Autodesk Fusion 360 part; units mm, degrees
note: some values were not read from the file. Set by a fixed rule: which sketch regions a step uses.
(part 8 of 20)
  spline S42 degree 5 poles (20.11, 20.9575) (20.11, 20.9576) (20.1102, 20.9577) (20.1104, 20.958) (20.1107, 20.9583) (20.1112, 20.9589) (20.1118, 20.9595) (20.1125, 20.9602) (20.1132, 20.961) (20.114, 20.9619) (20.1149, 20.9629) (20.1159, 20.9639) (20.1169, 20.9651) (20.118, 20.9663) (20.1192, 20.9675) (20.1204, 20.9689) (20.1217, 20.9704) (20.123, 20.9719) (20.1245, 20.9735) (20.126, 20.9752) (20.1275, 20.9769) (20.1291, 20.9787) (20.1308, 20.9806) (20.1325, 20.9826) (20.1343, 20.9847) (20.1361, 20.9868) (20.138, 20.989) (20.1399, 20.9912) (20.1419, 20.9936) (20.144, 20.996) (20.1461, 20.9984) (20.1482, 21.001) (20.1504, 21.0036) (20.1527, 21.0063) (20.155, 21.009) (20.1573, 21.0119) (20.1597, 21.0148) (20.1622, 21.0177) (20.1647, 21.0207) (20.1672, 21.0238) (20.1698, 21.027) (20.1724, 21.0302) (20.1751, 21.0335) (20.1778, 21.0368) (20.1806, 21.0403) (20.1834, 21.0437) (20.1862, 21.0473) (20.1891, 21.0509) (20.192, 21.0546) (20.195, 21.0583) (20.198, 21.0621) (20.201, 21.066) (20.2041, 21.0699) (20.2072, 21.0739) (20.2103, 21.0779) (20.2135, 21.082) (20.2167, 21.0862) (20.22, 21.0904) (20.2233, 21.0947) (20.2266, 21.099) (20.23, 21.1034) (20.2333, 21.1079) (20.2368, 21.1124) (20.2402, 21.117) (20.2437, 21.1216) (20.2472, 21.1263) (20.2508, 21.1311) (20.2544, 21.1359) (20.258, 21.1408) (20.2616, 21.1457) (20.2653, 21.1507) (20.269, 21.1557) (20.2727, 21.1608) (20.2765, 21.166) (20.2802, 21.1712) (20.2841, 21.1764) (20.2879, 21.1818) (20.2918, 21.1871) (20.2956, 21.1926) (20.2996, 21.1981) (20.3035, 21.2036) (20.3075, 21.2092) (20.3115, 21.2148) (20.3155, 21.2205) (20.3195, 21.2263) (20.3236, 21.2321) (20.3277, 21.238) (20.3318, 21.2439) (20.3359, 21.2498) (20.3401, 21.2559) (20.3442, 21.2619) (20.3484, 21.2681) (20.3527, 21.2742) (20.3569, 21.2805) (20.3612, 21.2867) (20.3655, 21.2931) (20.3698, 21.2995) (20.3741, 21.3059) (20.3784, 21.3124) (20.3828, 21.3189) (20.3872, 21.3255) (20.3916, 21.3321) (20.396, 21.3388) (20.4004, 21.3455) (20.4049, 21.3523) (20.4094, 21.3592) (20.4139, 21.3661) (20.4184, 21.373) (20.4229, 21.38) (20.4274, 21.387) (20.432, 21.3941) (20.4366, 21.4012) (20.4412, 21.4084) (20.4458, 21.4156) (20.4504, 21.4229) (20.455, 21.4302) (20.4597, 21.4376) (20.4644, 21.445) (20.469, 21.4525) (20.4737, 21.46) (20.4784, 21.4676) (20.4832, 21.4752) (20.4879, 21.4828) (20.4927, 21.4905) (20.4974, 21.4983) (20.5022, 21.5061) (20.507, 21.5139) (20.5118, 21.5218) (20.5166, 21.5297) (20.5214, 21.5377) (20.5263, 21.5458) (20.5311, 21.5538) (20.536, 21.5619) (20.5409, 21.5701) (20.5457, 21.5783) (20.5506, 21.5866) (20.5555, 21.5949) (20.5605, 21.6032) (20.5654, 21.6116) (20.5703, 21.6201) (20.5753, 21.6285) (20.5802, 21.6371) (20.5852, 21.6456) (20.5902, 21.6542) (20.5951, 21.6629) (20.6001, 21.6716) (20.6051, 21.6803) (20.6101, 21.6891) (20.6152, 21.698) (20.6202, 21.7068) (20.6252, 21.7158) (20.6303, 21.7247) (20.6353, 21.7337) (20.6404, 21.7428) (20.6454, 21.7519) (20.6505, 21.761) (20.6556, 21.7702) (20.6607, 21.7794) (20.6658, 21.7887) (20.6709, 21.798) (20.676, 21.8073) (20.6811, 21.8167) (20.6862, 21.8261) (20.6913, 21.8356) (20.6965, 21.8451) (20.7016, 21.8547) (20.7067, 21.8643) (20.7119, 21.8739) (20.717, 21.8836) (20.7222, 21.8933) (20.7274, 21.9031) (20.7325, 21.9129) (20.7377, 21.9228) (20.7429, 21.9326) (20.748, 21.9426) (20.7532, 21.9525) (20.7584, 21.9625) (20.7636, 21.9726) (20.7688, 21.9827) (20.774, 21.9928) (20.7792, 22.003) (20.7844, 22.0132) (20.7896, 22.0235) (20.7948, 22.0337) (20.8, 22.0441) (20.8052, 22.0544) (20.8105, 22.0649) (20.8157, 22.0753) (20.8209, 22.0858) (20.8261, 22.0963) (20.8313, 22.1069) (20.8366, 22.1175) (20.8418, 22.1281) (20.847, 22.1388) (20.8523, 22.1496) (20.8575, 22.1603) (20.8627, 22.1711) (20.868, 22.182) (20.8732, 22.1928) (20.8784, 22.2038) (20.8837, 22.2147) (20.8889, 22.2257) (20.8942, 22.2367) (20.8994, 22.2478) (20.9046, 22.2589) (20.9099, 22.2701) (20.9151, 22.2812) (20.9204, 22.2925) (20.9256, 22.3037) (20.9308, 22.315) (20.9361, 22.3264) (20.9413, 22.3377) (20.9466, 22.3491) (20.9518, 22.3606) (20.957, 22.3721) (20.9623, 22.3836) (20.9675, 22.3951) (20.9727, 22.4067) (20.978, 22.4184) (20.9832, 22.43) (20.9884, 22.4417) (20.9937, 22.4535) (20.9989, 22.4653) (21.0041, 22.4771) (21.0093, 22.4889) (21.0145, 22.5008) (21.0198, 22.5127) (21.025, 22.5247) (21.0302, 22.5367) (21.0354, 22.5487) (21.0406, 22.5608) (21.0458, 22.5729) (21.051, 22.585) (21.0562, 22.5972) (21.0614, 22.6094) (21.0666, 22.6217) (21.0718, 22.6339) (21.077, 22.6462) (21.0822, 22.6586) (21.0873, 22.671) (21.0925, 22.6834) (21.0967, 22.6934) (21.0998, 22.7009) (21.1018, 22.7059) (21.1029, 22.7084) knots 0 0 0 0 0 0 0.00416667 0.00833333 0.0125 0.01666667 0.02083333 0.025 0.02916667 0.03333333 0.0375 0.04166667 0.04583333 0.05 0.05416667 0.05833333 0.0625 0.06666667 0.07083333 0.075 0.07916667 0.08333333 0.0875 0.09166667 0.09583333 0.1 0.10416667 0.10833333 0.1125 0.11666667 0.12083333 0.125 0.12916667 0.13333333 0.1375 0.14166667 0.14583333 0.15 0.15416667 0.15833333 0.1625 0.16666667 0.17083333 0.175 0.17916667 0.18333333 0.1875 0.19166667 0.19583333 0.2 0.20416667 0.20833333 0.2125 0.21666667 0.22083333 0.225 0.22916667 0.23333333 0.2375 0.24166667 0.24583333 0.25 0.25416667 0.25833333 0.2625 0.26666667 0.27083333 0.275 0.27916667 0.28333333 0.2875 0.29166667 0.29583333 0.3 0.30416667 0.30833333 0.3125 0.31666667 0.32083333 0.325 0.32916667 0.33333333 0.3375 0.34166667 0.34583333 0.35 0.35416667 0.35833333 0.3625 0.36666667 0.37083333 0.375 0.37916667 0.38333333 0.3875 0.39166667 0.39583333 0.4 0.40416667 0.40833333 0.4125 0.41666667 0.42083333 0.425 0.42916667 0.43333333 0.4375 0.44166667 0.44583333 0.45 0.45416667 0.45833333 0.4625 0.46666667 0.47083333 0.475 0.47916667 0.48333333 0.4875 0.49166667 0.49583333 0.5 0.50416667 0.50833333 0.5125 0.51666667 0.52083333 0.525 0.52916667 0.53333333 0.5375 0.54166667 0.54583333 0.55 0.55416667 0.55833333 0.5625 0.56666667 0.57083333 0.575 0.57916667 0.58333333 0.5875 0.59166667 0.59583333 0.6 0.60416667 0.60833333 0.6125 0.61666667 0.62083333 0.625 0.62916667 0.63333333 0.6375 0.64166667 0.64583333 0.65 0.65416667 0.65833333 0.6625 0.66666667 0.67083333 0.675 0.67916667 0.68333333 0.6875 0.69166667 0.69583333 0.7 0.70416667 0.70833333 0.7125 0.71666667 0.72083333 0.725 0.72916667 0.73333333 0.7375 0.74166667 0.74583333 0.75 0.75416667 0.75833333 0.7625 0.76666667 0.77083333 0.775 0.77916667 0.78333333 0.7875 0.79166667 0.79583333 0.8 0.80416667 0.80833333 0.8125 0.81666667 0.82083333 0.825 0.82916667 0.83333333 0.8375 0.84166667 0.84583333 0.85 0.85416667 0.85833333 0.8625 0.86666667 0.87083333 0.875 0.87916667 0.88333333 0.8875 0.89166667 0.89583333 0.9 0.90416667 0.90833333 0.9125 0.91666667 0.92083333 0.925 0.92916667 0.93333333 0.9375 0.94166667 0.94583333 0.95 0.95416667 0.95833333 0.9625 0.96666667 0.97083333 0.975 0.97916667 0.98333333 0.9875 0.99166667 0.99583333 1 1 1 1 1 1
  spline S43 degree 5 poles (22.1904, 18.7406) (22.1905, 18.7407) (22.1907, 18.7408) (22.1909, 18.741) (22.1913, 18.7414) (22.1919, 18.7419) (22.1925, 18.7424) (22.1933, 18.7431) (22.1941, 18.7438) (22.195, 18.7446) (22.196, 18.7455) (22.197, 18.7464) (22.1982, 18.7474) (22.1994, 18.7485) (22.2007, 18.7497) (22.202, 18.7509) (22.2035, 18.7522) (22.205, 18.7536) (22.2066, 18.755) (22.2082, 18.7565) (22.2099, 18.7581) (22.2117, 18.7597) (22.2136, 18.7615) (22.2155, 18.7632) (22.2175, 18.7651) (22.2195, 18.767) (22.2216, 18.769) (22.2238, 18.771) (22.226, 18.7732) (22.2283, 18.7753) (22.2307, 18.7776) (22.2331, 18.7799) (22.2355, 18.7823) (22.238, 18.7847) (22.2406, 18.7872) (22.2433, 18.7897) (22.2459, 18.7924) (22.2487, 18.7951) (22.2515, 18.7978) (22.2543, 18.8006) (22.2572, 18.8035) (22.2602, 18.8064) (22.2632, 18.8094) (22.2662, 18.8124) (22.2693, 18.8156) (22.2725, 18.8187) (22.2757, 18.822) (22.2789, 18.8252) (22.2822, 18.8286) (22.2855, 18.832) (22.2889, 18.8355) (22.2923, 18.839) (22.2958, 18.8426) (22.2993, 18.8462) (22.3029, 18.8499) (22.3065, 18.8536) (22.3101, 18.8574) (22.3138, 18.8613) (22.3175, 18.8652) (22.3212, 18.8692) (22.325, 18.8732) (22.3289, 18.8773) (22.3328, 18.8814) (22.3367, 18.8856) (22.3406, 18.8899) (22.3446, 18.8942) (22.3486, 18.8986) (22.3527, 18.903) (22.3568, 18.9074) (22.3609, 18.9119) (22.3651, 18.9165) (22.3693, 18.9211) (22.3736, 18.9258) (22.3778, 18.9306) (22.3821, 18.9353) (22.3865, 18.9402) (22.3909, 18.9451) (22.3953, 18.95) (22.3997, 18.955) (22.4042, 18.96) (22.4087, 18.9651) (22.4132, 18.9703) (22.4177, 18.9755) (22.4223, 18.9807) (22.427, 18.986) (22.4316, 18.9914) (22.4363, 18.9968) (22.441, 19.0022) (22.4457, 19.0077) (22.4505, 19.0133) (22.4553, 19.0189) (22.4601, 19.0246) (22.4649, 19.0303) (22.4698, 19.036) (22.4747, 19.0418) (22.4796, 19.0477) (22.4846, 19.0536) (22.4895, 19.0595) (22.4945, 19.0655) (22.4996, 19.0715) (22.5046, 19.0776) (22.5097, 19.0838) (22.5148, 19.09) (22.5199, 19.0962) (22.525, 19.1025) (22.5302, 19.1088) (22.5354, 19.1152) (22.5406, 19.1216) (22.5458, 19.1281) (22.5511, 19.1346) (22.5564, 19.1412) (22.5617, 19.1478) (22.567, 19.1544) (22.5723, 19.1611) (22.5777, 19.1679) (22.583, 19.1747) (22.5884, 19.1815) (22.5939, 19.1884) (22.5993, 19.1954) (22.6048, 19.2024) (22.6102, 19.2094) (22.6157, 19.2165) (22.6212, 19.2236) (22.6268, 19.2307) (22.6323, 19.2379) (22.6379, 19.2452) (22.6435, 19.2525) (22.6491, 19.2598) (22.6547, 19.2672) (22.6603, 19.2747) (22.666, 19.2821) (22.6716, 19.2897) (22.6773, 19.2972) (22.683, 19.3048) (22.6887, 19.3125) (22.6945, 19.3202) (22.7002, 19.3279) (22.706, 19.3357) (22.7118, 19.3436) (22.7175, 19.3514) (22.7233, 19.3593) (22.7292, 19.3673) (22.735, 19.3753) (22.7408, 19.3834) (22.7467, 19.3914) (22.7526, 19.3996) (22.7585, 19.4078) (22.7644, 19.416) (22.7703, 19.4242) (22.7762, 19.4325) (22.7822, 19.4409) (22.7881, 19.4493) (22.7941, 19.4577) (22.8, 19.4662) (22.806, 19.4747) (22.812, 19.4832) (22.818, 19.4918) (22.8241, 19.5005) (22.8301, 19.5091) (22.8361, 19.5179) (22.8422, 19.5266) (22.8483, 19.5354) (22.8543, 19.5443) (22.8604, 19.5532) (22.8665, 19.5621) (22.8726, 19.5711) (22.8787, 19.5801) (22.8849, 19.5891) (22.891, 19.5982) (22.8971, 19.6073) (22.9033, 19.6165) (22.9095, 19.6257) (22.9156, 19.635) (22.9218, 19.6443) (22.928, 19.6536) (22.9342, 19.663) (22.9404, 19.6724) (22.9466, 19.6818) (22.9528, 19.6913) (22.9591, 19.7009) (22.9653, 19.7104) (22.9715, 19.72) (22.9778, 19.7297) (22.984, 19.7394) (22.9903, 19.7491) (22.9966, 19.7589) (23.0029, 19.7687) (23.0091, 19.7785) (23.0154, 19.7884) (23.0217, 19.7984) (23.028, 19.8083) (23.0343, 19.8183) (23.0406, 19.8284) (23.047, 19.8384) (23.0533, 19.8486) (23.0596, 19.8587) (23.066, 19.8689) (23.0723, 19.8791) (23.0786, 19.8894) (23.085, 19.8997) (23.0914, 19.9101) (23.0977, 19.9205) (23.1041, 19.9309) (23.1104, 19.9413) (23.1168, 19.9518) (23.1232, 19.9624) (23.1296, 19.973) (23.136, 19.9836) (23.1423, 19.9942) (23.1487, 20.0049) (23.1551, 20.0156) (23.1615, 20.0264) (23.1679, 20.0372) (23.1743, 20.048) (23.1807, 20.0589) (23.1872, 20.0698) (23.1936, 20.0808) (23.2, 20.0917) (23.2064, 20.1028) (23.2128, 20.1138) (23.2193, 20.1249) (23.2257, 20.136) (23.2321, 20.1472) (23.2385, 20.1584) (23.245, 20.1697) (23.2514, 20.1809) (23.2578, 20.1922) (23.2643, 20.2036) (23.2707, 20.215) (23.2771, 20.2264) (23.2836, 20.2379) (23.29, 20.2493) (23.2965, 20.2609) (23.3029, 20.2724) (23.3094, 20.284) (23.3158, 20.2957) (23.3222, 20.3073) (23.3287, 20.319) (23.3351, 20.3308) (23.3416, 20.3426) (23.348, 20.3544) (23.3532, 20.3639) (23.3571, 20.371) (23.3596, 20.3757) (23.3609, 20.3781) knots 0 0 0 0 0 0 0.00416667 0.00833333 0.0125 0.01666667 0.02083333 0.025 0.02916667 0.03333333 0.0375 0.04166667 0.04583333 0.05 0.05416667 0.05833333 0.0625 0.06666667 0.07083333 0.075 0.07916667 0.08333333 0.0875 0.09166667 0.09583333 0.1 0.10416667 0.10833333 0.1125 0.11666667 0.12083333 0.125 0.12916667 0.13333333 0.1375 0.14166667 0.14583333 0.15 0.15416667 0.15833333 0.1625 0.16666667 0.17083333 0.175 0.17916667 0.18333333 0.1875 0.19166667 0.19583333 0.2 0.20416667 0.20833333 0.2125 0.21666667 0.22083333 0.225 0.22916667 0.23333333 0.2375 0.24166667 0.24583333 0.25 0.25416667 0.25833333 0.2625 0.26666667 0.27083333 0.275 0.27916667 0.28333333 0.2875 0.29166667 0.29583333 0.3 0.30416667 0.30833333 0.3125 0.31666667 0.32083333 0.325 0.32916667 0.33333333 0.3375 0.34166667 0.34583333 0.35 0.35416667 0.35833333 0.3625 0.36666667 0.37083333 0.375 0.37916667 0.38333333 0.3875 0.39166667 0.39583333 0.4 0.40416667 0.40833333 0.4125 0.41666667 0.42083333 0.425 0.42916667 0.43333333 0.4375 0.44166667 0.44583333 0.45 0.45416667 0.45833333 0.4625 0.46666667 0.47083333 0.475 0.47916667 0.48333333 0.4875 0.49166667 0.49583333 0.5 0.50416667 0.50833333 0.5125 0.51666667 0.52083333 0.525 0.52916667 0.53333333 0.5375 0.54166667 0.54583333 0.55 0.55416667 0.55833333 0.5625 0.56666667 0.57083333 0.575 0.57916667 0.58333333 0.5875 0.59166667 0.59583333 0.6 0.60416667 0.60833333 0.6125 0.61666667 0.62083333 0.625 0.62916667 0.63333333 0.6375 0.64166667 0.64583333 0.65 0.65416667 0.65833333 0.6625 0.66666667 0.67083333 0.675 0.67916667 0.68333333 0.6875 0.69166667 0.69583333 0.7 0.70416667 0.70833333 0.7125 0.71666667 0.72083333 0.725 0.72916667 0.73333333 0.7375 0.74166667 0.74583333 0.75 0.75416667 0.75833333 0.7625 0.76666667 0.77083333 0.775 0.77916667 0.78333333 0.7875 0.79166667 0.79583333 0.8 0.80416667 0.80833333 0.8125 0.81666667 0.82083333 0.825 0.82916667 0.83333333 0.8375 0.84166667 0.84583333 0.85 0.85416667 0.85833333 0.8625 0.86666667 0.87083333 0.875 0.87916667 0.88333333 0.8875 0.89166667 0.89583333 0.9 0.90416667 0.90833333 0.9125 0.91666667 0.92083333 0.925 0.92916667 0.93333333 0.9375 0.94166667 0.94583333 0.95 0.95416667 0.95833333 0.9625 0.96666667 0.97083333 0.975 0.97916667 0.98333333 0.9875 0.99166667 0.99583333 1 1 1 1 1 1
  spline S44 degree 5 poles (29.0307, -0.9213) (29.0307, -0.9213) (29.0309, -0.9213) (29.0313, -0.9213) (29.0318, -0.9213) (29.0325, -0.9213) (29.0334, -0.9213) (29.0344, -0.9214) (29.0355, -0.9214) (29.0367, -0.9214) (29.038, -0.9214) (29.0394, -0.9214) (29.0409, -0.9214) (29.0425, -0.9214) (29.0443, -0.9214) (29.0461, -0.9214) (29.0481, -0.9214) (29.0501, -0.9214) (29.0522, -0.9214) (29.0545, -0.9214) (29.0568, -0.9214) (29.0592, -0.9213) (29.0618, -0.9213) (29.0644, -0.9212) (29.0671, -0.9212) (29.0699, -0.9211) (29.0728, -0.9211) (29.0758, -0.921) (29.0788, -0.9209) (29.082, -0.9208) (29.0852, -0.9208) (29.0886, -0.9206) (29.092, -0.9205) (29.0955, -0.9204) (29.0991, -0.9203) (29.1028, -0.9201) (29.1065, -0.92) (29.1103, -0.9198) (29.1143, -0.9197) (29.1183, -0.9195) (29.1223, -0.9193) (29.1265, -0.9191) (29.1307, -0.9189) (29.135, -0.9186) (29.1394, -0.9184) (29.1439, -0.9182) (29.1484, -0.9179) (29.153, -0.9176) (29.1577, -0.9173) (29.1624, -0.917) (29.1673, -0.9167) (29.1722, -0.9164) (29.1771, -0.9161) (29.1822, -0.9157) (29.1873, -0.9153) (29.1925, -0.915) (29.1977, -0.9146) (29.203, -0.9141) (29.2084, -0.9137) (29.2139, -0.9133) (29.2194, -0.9128) (29.225, -0.9124) (29.2306, -0.9119) (29.2363, -0.9114) (29.2421, -0.9109) (29.248, -0.9103) (29.2539, -0.9098) (29.2599, -0.9092) (29.2659, -0.9087) (29.272, -0.9081) (29.2781, -0.9075) (29.2844, -0.9068) (29.2906, -0.9062) (29.297, -0.9055) (29.3034, -0.9049) (29.3099, -0.9042) (29.3164, -0.9035) (29.323, -0.9027) (29.3296, -0.902) (29.3363, -0.9012) (29.343, -0.9005) (29.3498, -0.8997) (29.3567, -0.8989) (29.3636, -0.898) (29.3706, -0.8972) (29.3777, -0.8963) (29.3847, -0.8954) (29.3919, -0.8945) (29.3991, -0.8936) (29.4063, -0.8927) (29.4137, -0.8917) (29.421, -0.8907) (29.4284, -0.8897) (29.4359, -0.8887) (29.4434, -0.8877) (29.451, -0.8866) (29.4586, -0.8856) (29.4663, -0.8845) (29.474, -0.8834) (29.4818, -0.8822) (29.4896, -0.8811) (29.4975, -0.8799) (29.5054, -0.8787) (29.5134, -0.8775) (29.5214, -0.8763) (29.5295, -0.875) (29.5376, -0.8738) (29.5458, -0.8725) (29.554, -0.8712) (29.5623, -0.8698) (29.5706, -0.8685) (29.5789, -0.8671) (29.5873, -0.8657) (29.5958, -0.8643) (29.6043, -0.8629) (29.6128, -0.8614) (29.6214, -0.86) (29.6301, -0.8585) (29.6388, -0.8569) (29.6475, -0.8554) (29.6563, -0.8538) (29.6651, -0.8523) (29.6739, -0.8507) (29.6828, -0.849) (29.6918, -0.8474) (29.7008, -0.8457) (29.7098, -0.844) (29.7189, -0.8423) (29.728, -0.8406) (29.7372, -0.8388) (29.7464, -0.8371) (29.7556, -0.8353) (29.7649, -0.8334) (29.7742, -0.8316) (29.7836, -0.8297) (29.793, -0.8279) (29.8025, -0.8259) (29.812, -0.824) (29.8215, -0.8221) (29.8311, -0.8201) (29.8407, -0.8181) (29.8503, -0.8161) (29.86, -0.814) (29.8697, -0.812) (29.8795, -0.8099) (29.8893, -0.8078) (29.8992, -0.8056) (29.909, -0.8035) (29.919, -0.8013) (29.9289, -0.7991) (29.9389, -0.7969) (29.949, -0.7946) (29.959, -0.7923) (29.9691, -0.79) (29.9793, -0.7877) (29.9895, -0.7854) (29.9997, -0.783) (30.0099, -0.7806) (30.0202, -0.7782) (30.0306, -0.7758) (30.0409, -0.7733) (30.0513, -0.7708) (30.0618, -0.7683) (30.0722, -0.7658) (30.0827, -0.7632) (30.0933, -0.7606) (30.1038, -0.758) (30.1145, -0.7554) (30.1251, -0.7528) (30.1358, -0.7501) (30.1465, -0.7474) (30.1572, -0.7447) (30.168, -0.7419) (30.1788, -0.7391) (30.1897, -0.7364) (30.2005, -0.7335) (30.2114, -0.7307) (30.2224, -0.7278) (30.2334, -0.7249) (30.2444, -0.722) (30.2554, -0.7191) (30.2665, -0.7161) (30.2776, -0.7131) (30.2887, -0.7101) (30.2999, -0.7071) (30.3111, -0.704) (30.3223, -0.7009) (30.3336, -0.6978) (30.3448, -0.6947) (30.3562, -0.6915) (30.3675, -0.6883) (30.3789, -0.6851) (30.3903, -0.6819) (30.4017, -0.6786) (30.4132, -0.6753) (30.4247, -0.672) (30.4362, -0.6687) (30.4478, -0.6653) (30.4594, -0.6619) (30.471, -0.6585) (30.4827, -0.6551) (30.4943, -0.6516) (30.506, -0.6481) (30.5178, -0.6446) (30.5295, -0.6411) (30.5413, -0.6375) (30.5531, -0.6339) (30.565, -0.6303) (30.5769, -0.6267) (30.5888, -0.623) (30.6007, -0.6193) (30.6126, -0.6156) (30.6246, -0.6118) (30.6366, -0.6081) (30.6487, -0.6043) (30.6607, -0.6005) (30.6728, -0.5966) (30.685, -0.5927) (30.6971, -0.5889) (30.7093, -0.5849) (30.7215, -0.581) (30.7337, -0.577) (30.7459, -0.573) (30.7582, -0.569) (30.7705, -0.5649) (30.7828, -0.5609) (30.7952, -0.5568) (30.8076, -0.5526) (30.82, -0.5485) (30.8324, -0.5443) (30.8448, -0.5401) (30.8573, -0.5359) (30.8698, -0.5316) (30.8823, -0.5273) (30.8949, -0.523) (30.9075, -0.5187) (30.9201, -0.5143) (30.9327, -0.5099) (30.9453, -0.5055) (30.958, -0.5011) (30.9707, -0.4966) (30.9809, -0.493) (30.9885, -0.4903) (30.9936, -0.4885) (30.9962, -0.4876) knots 0 0 0 0 0 0 0.00416667 0.00833333 0.0125 0.01666667 0.02083333 0.025 0.02916667 0.03333333 0.0375 0.04166667 0.04583333 0.05 0.05416667 0.05833333 0.0625 0.06666667 0.07083333 0.075 0.07916667 0.08333333 0.0875 0.09166667 0.09583333 0.1 0.10416667 0.10833333 0.1125 0.11666667 0.12083333 0.125 0.12916667 0.13333333 0.1375 0.14166667 0.14583333 0.15 0.15416667 0.15833333 0.1625 0.16666667 0.17083333 0.175 0.17916667 0.18333333 0.1875 0.19166667 0.19583333 0.2 0.20416667 0.20833333 0.2125 0.21666667 0.22083333 0.225 0.22916667 0.23333333 0.2375 0.24166667 0.24583333 0.25 0.25416667 0.25833333 0.2625 0.26666667 0.27083333 0.275 0.27916667 0.28333333 0.2875 0.29166667 0.29583333 0.3 0.30416667 0.30833333 0.3125 0.31666667 0.32083333 0.325 0.32916667 0.33333333 0.3375 0.34166667 0.34583333 0.35 0.35416667 0.35833333 0.3625 0.36666667 0.37083333 0.375 0.37916667 0.38333333 0.3875 0.39166667 0.39583333 0.4 0.40416667 0.40833333 0.4125 0.41666667 0.42083333 0.425 0.42916667 0.43333333 0.4375 0.44166667 0.44583333 0.45 0.45416667 0.45833333 0.4625 0.46666667 0.47083333 0.475 0.47916667 0.48333333 0.4875 0.49166667 0.49583333 0.5 0.50416667 0.50833333 0.5125 0.51666667 0.52083333 0.525 0.52916667 0.53333333 0.5375 0.54166667 0.54583333 0.55 0.55416667 0.55833333 0.5625 0.56666667 0.57083333 0.575 0.57916667 0.58333333 0.5875 0.59166667 0.59583333 0.6 0.60416667 0.60833333 0.6125 0.61666667 0.62083333 0.625 0.62916667 0.63333333 0.6375 0.64166667 0.64583333 0.65 0.65416667 0.65833333 0.6625 0.66666667 0.67083333 0.675 0.67916667 0.68333333 0.6875 0.69166667 0.69583333 0.7 0.70416667 0.70833333 0.7125 0.71666667 0.72083333 0.725 0.72916667 0.73333333 0.7375 0.74166667 0.74583333 0.75 0.75416667 0.75833333 0.7625 0.76666667 0.77083333 0.775 0.77916667 0.78333333 0.7875 0.79166667 0.79583333 0.8 0.80416667 0.80833333 0.8125 0.81666667 0.82083333 0.825 0.82916667 0.83333333 0.8375 0.84166667 0.84583333 0.85 0.85416667 0.85833333 0.8625 0.86666667 0.87083333 0.875 0.87916667 0.88333333 0.8875 0.89166667 0.89583333 0.9 0.90416667 0.90833333 0.9125 0.91666667 0.92083333 0.925 0.92916667 0.93333333 0.9375 0.94166667 0.94583333 0.95 0.95416667 0.95833333 0.9625 0.96666667 0.97083333 0.975 0.97916667 0.98333333 0.9875 0.99166667 0.99583333 1 1 1 1 1 1
  arc A46 (18.5501, 21.9649) -> (17.6281, 22.7115) centre (0, 0) ccw
  spline S45 degree 5 poles (-30.9962, -0.4876) (-30.9936, -0.4885) (-30.9885, -0.4903) (-30.9809, -0.493) (-30.9707, -0.4966) (-30.958, -0.5011) (-30.9453, -0.5055) (-30.9327, -0.5099) (-30.9201, -0.5143) (-30.9075, -0.5187) (-30.8949, -0.523) (-30.8823, -0.5273) (-30.8698, -0.5316) (-30.8573, -0.5359) (-30.8448, -0.5401) (-30.8324, -0.5443) (-30.82, -0.5485) (-30.8076, -0.5526) (-30.7952, -0.5568) (-30.7828, -0.5609) (-30.7705, -0.5649) (-30.7582, -0.569) (-30.7459, -0.573) (-30.7337, -0.577) (-30.7215, -0.581) (-30.7093, -0.5849) (-30.6971, -0.5889) (-30.685, -0.5927) (-30.6728, -0.5966) (-30.6607, -0.6005) (-30.6487, -0.6043) (-30.6366, -0.6081) (-30.6246, -0.6118) (-30.6126, -0.6156) (-30.6007, -0.6193) (-30.5888, -0.623) (-30.5769, -0.6267) (-30.565, -0.6303) (-30.5531, -0.6339) (-30.5413, -0.6375) (-30.5295, -0.6411) (-30.5178, -0.6446) (-30.506, -0.6481) (-30.4943, -0.6516) (-30.4827, -0.6551) (-30.471, -0.6585) (-30.4594, -0.6619) (-30.4478, -0.6653) (-30.4362, -0.6687) (-30.4247, -0.672) (-30.4132, -0.6753) (-30.4017, -0.6786) (-30.3903, -0.6819) (-30.3789, -0.6851) (-30.3675, -0.6883) (-30.3562, -0.6915) (-30.3448, -0.6947) (-30.3336, -0.6978) (-30.3223, -0.7009) (-30.3111, -0.704) (-30.2999, -0.7071) (-30.2887, -0.7101) (-30.2776, -0.7131) (-30.2665, -0.7161) (-30.2554, -0.7191) (-30.2444, -0.722) (-30.2334, -0.7249) (-30.2224, -0.7278) (-30.2114, -0.7307) (-30.2005, -0.7335) (-30.1897, -0.7364) (-30.1788, -0.7391) (-30.168, -0.7419) (-30.1572, -0.7447) (-30.1465, -0.7474) (-30.1358, -0.7501) (-30.1251, -0.7528) (-30.1145, -0.7554) (-30.1038, -0.758) (-30.0933, -0.7606) (-30.0827, -0.7632) (-30.0722, -0.7658) (-30.0618, -0.7683) (-30.0513, -0.7708) (-30.0409, -0.7733) (-30.0306, -0.7758) (-30.0202, -0.7782) (-30.0099, -0.7806) (-29.9997, -0.783) (-29.9895, -0.7854) (-29.9793, -0.7877) (-29.9691, -0.79) (-29.959, -0.7923) (-29.949, -0.7946) (-29.9389, -0.7969) (-29.9289, -0.7991) (-29.919, -0.8013) (-29.909, -0.8035) (-29.8992, -0.8056) (-29.8893, -0.8078) (-29.8795, -0.8099) (-29.8697, -0.812) (-29.86, -0.814) (-29.8503, -0.8161) (-29.8407, -0.8181) (-29.8311, -0.8201) (-29.8215, -0.8221) (-29.812, -0.824) (-29.8025, -0.8259) (-29.793, -0.8279) (-29.7836, -0.8297) (-29.7742, -0.8316) (-29.7649, -0.8334) (-29.7556, -0.8353) (-29.7464, -0.8371) (-29.7372, -0.8388) (-29.728, -0.8406) (-29.7189, -0.8423) (-29.7098, -0.844) (-29.7008, -0.8457) (-29.6918, -0.8474) (-29.6828, -0.849) (-29.6739, -0.8507) (-29.6651, -0.8523) (-29.6563, -0.8538) (-29.6475, -0.8554) (-29.6388, -0.8569) (-29.6301, -0.8585) (-29.6214, -0.86) (-29.6128, -0.8614) (-29.6043, -0.8629) (-29.5958, -0.8643) (-29.5873, -0.8657) (-29.5789, -0.8671) (-29.5706, -0.8685) (-29.5623, -0.8698) (-29.554, -0.8712) (-29.5458, -0.8725) (-29.5376, -0.8738) (-29.5295, -0.875) (-29.5214, -0.8763) (-29.5134, -0.8775) (-29.5054, -0.8787) (-29.4975, -0.8799) (-29.4896, -0.8811) (-29.4818, -0.8822) (-29.474, -0.8834) (-29.4663, -0.8845) (-29.4586, -0.8856) (-29.451, -0.8866) (-29.4434, -0.8877) (-29.4359, -0.8887) (-29.4284, -0.8897) (-29.421, -0.8907) (-29.4137, -0.8917) (-29.4063, -0.8927) (-29.3991, -0.8936) (-29.3919, -0.8945) (-29.3847, -0.8954) (-29.3777, -0.8963) (-29.3706, -0.8972) (-29.3636, -0.898) (-29.3567, -0.8989) (-29.3498, -0.8997) (-29.343, -0.9005) (-29.3363, -0.9012) (-29.3296, -0.902) (-29.323, -0.9027) (-29.3164, -0.9035) (-29.3099, -0.9042) (-29.3034, -0.9049) (-29.297, -0.9055) (-29.2906, -0.9062) (-29.2844, -0.9068) (-29.2781, -0.9075) (-29.272, -0.9081) (-29.2659, -0.9087) (-29.2599, -0.9092) (-29.2539, -0.9098) (-29.248, -0.9103) (-29.2421, -0.9109) (-29.2363, -0.9114) (-29.2306, -0.9119) (-29.225, -0.9124) (-29.2194, -0.9128) (-29.2139, -0.9133) (-29.2084, -0.9137) (-29.203, -0.9141) (-29.1977, -0.9146) (-29.1925, -0.915) (-29.1873, -0.9153) (-29.1822, -0.9157) (-29.1771, -0.9161) (-29.1722, -0.9164) (-29.1673, -0.9167) (-29.1624, -0.917) (-29.1577, -0.9173) (-29.153, -0.9176) (-29.1484, -0.9179) (-29.1439, -0.9182) (-29.1394, -0.9184) (-29.135, -0.9186) (-29.1307, -0.9189) (-29.1265, -0.9191) (-29.1223, -0.9193) (-29.1183, -0.9195) (-29.1143, -0.9197) (-29.1103, -0.9198) (-29.1065, -0.92) (-29.1028, -0.9201) (-29.0991, -0.9203) (-29.0955, -0.9204) (-29.092, -0.9205) (-29.0886, -0.9206) (-29.0852, -0.9208) (-29.082, -0.9208) (-29.0788, -0.9209) (-29.0758, -0.921) (-29.0728, -0.9211) (-29.0699, -0.9211) (-29.0671, -0.9212) (-29.0644, -0.9212) (-29.0618, -0.9213) (-29.0592, -0.9213) (-29.0568, -0.9214) (-29.0545, -0.9214) (-29.0522, -0.9214) (-29.0501, -0.9214) (-29.0481, -0.9214) (-29.0461, -0.9214) (-29.0443, -0.9214) (-29.0425, -0.9214) (-29.0409, -0.9214) (-29.0394, -0.9214) (-29.038, -0.9214) (-29.0367, -0.9214) (-29.0355, -0.9214) (-29.0344, -0.9214) (-29.0334, -0.9213) (-29.0325, -0.9213) (-29.0318, -0.9213) (-29.0313, -0.9213) (-29.0309, -0.9213) (-29.0307, -0.9213) (-29.0307, -0.9213) knots -1 -1 -1 -1 -1 -1 -0.99583333 -0.99166667 -0.9875 -0.98333333 -0.97916667 -0.975 -0.97083333 -0.96666667 -0.9625 -0.95833333 -0.95416667 -0.95 -0.94583333 -0.94166667 -0.9375 -0.93333333 -0.92916667 -0.925 -0.92083333 -0.91666667 -0.9125 -0.90833333 -0.90416667 -0.9 -0.89583333 -0.89166667 -0.8875 -0.88333333 -0.87916667 -0.875 -0.87083333 -0.86666667 -0.8625 -0.85833333 -0.85416667 -0.85 -0.84583333 -0.84166667 -0.8375 -0.83333333 -0.82916667 -0.825 -0.82083333 -0.81666667 -0.8125 -0.80833333 -0.80416667 -0.8 -0.79583333 -0.79166667 -0.7875 -0.78333333 -0.77916667 -0.775 -0.77083333 -0.76666667 -0.7625 -0.75833333 -0.75416667 -0.75 -0.74583333 -0.74166667 -0.7375 -0.73333333 -0.72916667 -0.725 -0.72083333 -0.71666667 -0.7125 -0.70833333 -0.70416667 -0.7 -0.69583333 -0.69166667 -0.6875 -0.68333333 -0.67916667 -0.675 -0.67083333 -0.66666667 -0.6625 -0.65833333 -0.65416667 -0.65 -0.64583333 -0.64166667 -0.6375 -0.63333333 -0.62916667 -0.625 -0.62083333 -0.61666667 -0.6125 -0.60833333 -0.60416667 -0.6 -0.59583333 -0.59166667 -0.5875 -0.58333333 -0.57916667 -0.575 -0.57083333 -0.56666667 -0.5625 -0.55833333 -0.55416667 -0.55 -0.54583333 -0.54166667 -0.5375 -0.53333333 -0.52916667 -0.525 -0.52083333 -0.51666667 -0.5125 -0.50833333 -0.50416667 -0.5 -0.49583333 -0.49166667 -0.4875 -0.48333333 -0.47916667 -0.475 -0.47083333 -0.46666667 -0.4625 -0.45833333 -0.45416667 -0.45 -0.44583333 -0.44166667 -0.4375 -0.43333333 -0.42916667 -0.425 -0.42083333 -0.41666667 -0.4125 -0.40833333 -0.40416667 -0.4 -0.39583333 -0.39166667 -0.3875 -0.38333333 -0.37916667 -0.375 -0.37083333 -0.36666667 -0.3625 -0.35833333 -0.35416667 -0.35 -0.34583333 -0.34166667 -0.3375 -0.33333333 -0.32916667 -0.325 -0.32083333 -0.31666667 -0.3125 -0.30833333 -0.30416667 -0.3 -0.29583333 -0.29166667 -0.2875 -0.28333333 -0.27916667 -0.275 -0.27083333 -0.26666667 -0.2625 -0.25833333 -0.25416667 -0.25 -0.24583333 -0.24166667 -0.2375 -0.23333333 -0.22916667 -0.225 -0.22083333 -0.21666667 -0.2125 -0.20833333 -0.20416667 -0.2 -0.19583333 -0.19166667 -0.1875 -0.18333333 -0.17916667 -0.175 -0.17083333 -0.16666667 -0.1625 -0.15833333 -0.15416667 -0.15 -0.14583333 -0.14166667 -0.1375 -0.13333333 -0.12916667 -0.125 -0.12083333 -0.11666667 -0.1125 -0.10833333 -0.10416667 -0.1 -0.09583333 -0.09166667 -0.0875 -0.08333333 -0.07916667 -0.075 -0.07083333 -0.06666667 -0.0625 -0.05833333 -0.05416667 -0.05 -0.04583333 -0.04166667 -0.0375 -0.03333333 -0.02916667 -0.025 -0.02083333 -0.01666667 -0.0125 -0.00833333 -0.00416667 0 0 0 0 0 0
  arc A47 (-28.4828, -3.9106) -> (-28.2972, -5.0824) centre (0, 0) ccw
  line L100 (-28.2972, -5.0824) -> (-28.587, -5.1345)
  arc A48 (-28.7355, -0.9119) -> (-28.6734, -2.0967) centre (0, 0) ccw
  arc A49 (-30.8773, -2.755) -> (-30.7754, -3.7249) centre (0, 0) ccw
  spline S46 degree 5 poles (27.3251, -9.8472) (27.3252, -9.8472) (27.3254, -9.8473) (27.3257, -9.8474) (27.3262, -9.8475) (27.3269, -9.8478) (27.3277, -9.8481) (27.3286, -9.8484) (27.3296, -9.8487) (27.3308, -9.8491) (27.332, -9.8495) (27.3334, -9.85) (27.3348, -9.8505) (27.3364, -9.851) (27.338, -9.8515) (27.3398, -9.8521) (27.3416, -9.8527) (27.3435, -9.8533) (27.3456, -9.8539) (27.3477, -9.8546) (27.3499, -9.8553) (27.3523, -9.856) (27.3547, -9.8568) (27.3572, -9.8575) (27.3598, -9.8583) (27.3625, -9.8591) (27.3652, -9.86) (27.3681, -9.8608) (27.371, -9.8617) (27.3741, -9.8626) (27.3772, -9.8635) (27.3804, -9.8645) (27.3837, -9.8654) (27.387, -9.8664) (27.3905, -9.8674) (27.394, -9.8684) (27.3976, -9.8694) (27.4013, -9.8704) (27.4051, -9.8715) (27.409, -9.8725) (27.4129, -9.8736) (27.4169, -9.8747) (27.421, -9.8758) (27.4252, -9.8769) (27.4294, -9.878) (27.4337, -9.8792) (27.4381, -9.8803) (27.4426, -9.8815) (27.4471, -9.8827) (27.4517, -9.8838) (27.4564, -9.885) (27.4612, -9.8862) (27.466, -9.8874) (27.4709, -9.8887) (27.4759, -9.8899) (27.481, -9.8911) (27.4861, -9.8924) (27.4912, -9.8936) (27.4965, -9.8949) (27.5018, -9.8962) (27.5072, -9.8974) (27.5127, -9.8987) (27.5182, -9.9) (27.5238, -9.9013) (27.5294, -9.9026) (27.5352, -9.9039) (27.5409, -9.9052) (27.5468, -9.9065) (27.5527, -9.9079) (27.5587, -9.9092) (27.5647, -9.9105) (27.5709, -9.9118) (27.577, -9.9132) (27.5833, -9.9145) (27.5896, -9.9158) (27.5959, -9.9172) (27.6023, -9.9185) (27.6088, -9.9199) (27.6154, -9.9212) (27.622, -9.9225) (27.6286, -9.9239) (27.6353, -9.9252) (27.6421, -9.9266) (27.649, -9.9279) (27.6559, -9.9293) (27.6628, -9.9306) (27.6698, -9.932) (27.6769, -9.9333) (27.6841, -9.9347) (27.6912, -9.936) (27.6985, -9.9374) (27.7058, -9.9387) (27.7132, -9.9401) (27.7206, -9.9414) (27.728, -9.9428) (27.7356, -9.9441) (27.7431, -9.9454) (27.7508, -9.9468) (27.7585, -9.9481) (27.7662, -9.9494) (27.774, -9.9508) (27.7819, -9.9521) (27.7898, -9.9534) (27.7977, -9.9547) (27.8057, -9.956) (27.8138, -9.9573) (27.8219, -9.9586) (27.8301, -9.9599) (27.8383, -9.9612) (27.8466, -9.9625) (27.8549, -9.9638) (27.8633, -9.9651) (27.8717, -9.9664) (27.8802, -9.9676) (27.8887, -9.9689) (27.8973, -9.9701) (27.9059, -9.9714) (27.9146, -9.9726) (27.9233, -9.9739) (27.9321, -9.9751) (27.9409, -9.9763) (27.9498, -9.9776) (27.9587, -9.9788) (27.9677, -9.98) (27.9767, -9.9812) (27.9858, -9.9824) (27.9949, -9.9836) (28.004, -9.9847) (28.0133, -9.9859) (28.0225, -9.9871) (28.0318, -9.9882) (28.0412, -9.9894) (28.0506, -9.9905) (28.06, -9.9916) (28.0695, -9.9928) (28.079, -9.9939) (28.0886, -9.995) (28.0982, -9.9961) (28.1079, -9.9972) (28.1176, -9.9983) (28.1274, -9.9993) (28.1372, -10.0004) (28.147, -10.0014) (28.1569, -10.0025) (28.1668, -10.0035) (28.1768, -10.0045) (28.1868, -10.0055) (28.1969, -10.0065) (28.207, -10.0075) (28.2172, -10.0085) (28.2274, -10.0095) (28.2376, -10.0104) (28.2479, -10.0114) (28.2582, -10.0123) (28.2686, -10.0133) (28.279, -10.0142) (28.2894, -10.0151) (28.2999, -10.016) (28.3105, -10.0169) (28.321, -10.0177) (28.3317, -10.0186) (28.3423, -10.0195) (28.353, -10.0203) (28.3638, -10.0211) (28.3745, -10.0219) (28.3854, -10.0227) (28.3962, -10.0235) (28.4071, -10.0243) (28.4181, -10.0251) (28.429, -10.0258) (28.44, -10.0266) (28.4511, -10.0273) (28.4622, -10.028) (28.4733, -10.0287) (28.4845, -10.0294) (28.4957, -10.0301) (28.507, -10.0308) (28.5183, -10.0314) (28.5296, -10.0321) (28.541, -10.0327) (28.5524, -10.0333) (28.5638, -10.0339) (28.5753, -10.0345) (28.5868, -10.0351) (28.5984, -10.0356) (28.61, -10.0362) (28.6216, -10.0367) (28.6333, -10.0372) (28.645, -10.0377) (28.6567, -10.0382) (28.6685, -10.0387) (28.6803, -10.0392) (28.6922, -10.0396) (28.7041, -10.04) (28.716, -10.0405) (28.728, -10.0409) (28.74, -10.0412) (28.752, -10.0416) (28.7641, -10.042) (28.7762, -10.0423) (28.7883, -10.0427) (28.8005, -10.043) (28.8127, -10.0433) (28.8249, -10.0436) (28.8372, -10.0438) (28.8495, -10.0441) (28.8619, -10.0443) (28.8743, -10.0445) (28.8867, -10.0448) (28.8991, -10.0449) (28.9116, -10.0451) (28.9241, -10.0453) (28.9367, -10.0454) (28.9493, -10.0456) (28.9619, -10.0457) (28.9745, -10.0458) (28.9872, -10.0458) (29, -10.0459) (29.0127, -10.046) (29.0255, -10.046) (29.0383, -10.046) (29.0512, -10.046) (29.0641, -10.046) (29.077, -10.046) (29.0899, -10.0459) (29.1029, -10.0458) (29.1159, -10.0458) (29.129, -10.0457) (29.142, -10.0455) (29.1551, -10.0454) (29.1683, -10.0453) (29.1815, -10.0451) (29.1947, -10.0449) (29.2079, -10.0447) (29.2212, -10.0445) (29.2345, -10.0442) (29.2478, -10.044) (29.2612, -10.0437) (29.2745, -10.0434) (29.288, -10.0431) (29.3014, -10.0428) (29.3122, -10.0425) (29.3203, -10.0423) (29.3257, -10.0422) (29.3284, -10.0421) knots 0 0 0 0 0 0 0.00416667 0.00833333 0.0125 0.01666667 0.02083333 0.025 0.02916667 0.03333333 0.0375 0.04166667 0.04583333 0.05 0.05416667 0.05833333 0.0625 0.06666667 0.07083333 0.075 0.07916667 0.08333333 0.0875 0.09166667 0.09583333 0.1 0.10416667 0.10833333 0.1125 0.11666667 0.12083333 0.125 0.12916667 0.13333333 0.1375 0.14166667 0.14583333 0.15 0.15416667 0.15833333 0.1625 0.16666667 0.17083333 0.175 0.17916667 0.18333333 0.1875 0.19166667 0.19583333 0.2 0.20416667 0.20833333 0.2125 0.21666667 0.22083333 0.225 0.22916667 0.23333333 0.2375 0.24166667 0.24583333 0.25 0.25416667 0.25833333 0.2625 0.26666667 0.27083333 0.275 0.27916667 0.28333333 0.2875 0.29166667 0.29583333 0.3 0.30416667 0.30833333 0.3125 0.31666667 0.32083333 0.325 0.32916667 0.33333333 0.3375 0.34166667 0.34583333 0.35 0.35416667 0.35833333 0.3625 0.36666667 0.37083333 0.375 0.37916667 0.38333333 0.3875 0.39166667 0.39583333 0.4 0.40416667 0.40833333 0.4125 0.41666667 0.42083333 0.425 0.42916667 0.43333333 0.4375 0.44166667 0.44583333 0.45 0.45416667 0.45833333 0.4625 0.46666667 0.47083333 0.475 0.47916667 0.48333333 0.4875 0.49166667 0.49583333 0.5 0.50416667 0.50833333 0.5125 0.51666667 0.52083333 0.525 0.52916667 0.53333333 0.5375 0.54166667 0.54583333 0.55 0.55416667 0.55833333 0.5625 0.56666667 0.57083333 0.575 0.57916667 0.58333333 0.5875 0.59166667 0.59583333 0.6 0.60416667 0.60833333 0.6125 0.61666667 0.62083333 0.625 0.62916667 0.63333333 0.6375 0.64166667 0.64583333 0.65 0.65416667 0.65833333 0.6625 0.66666667 0.67083333 0.675 0.67916667 0.68333333 0.6875 0.69166667 0.69583333 0.7 0.70416667 0.70833333 0.7125 0.71666667 0.72083333 0.725 0.72916667 0.73333333 0.7375 0.74166667 0.74583333 0.75 0.75416667 0.75833333 0.7625 0.76666667 0.77083333 0.775 0.77916667 0.78333333 0.7875 0.79166667 0.79583333 0.8 0.80416667 0.80833333 0.8125 0.81666667 0.82083333 0.825 0.82916667 0.83333333 0.8375 0.84166667 0.84583333 0.85 0.85416667 0.85833333 0.8625 0.86666667 0.87083333 0.875 0.87916667 0.88333333 0.8875 0.89166667 0.89583333 0.9 0.90416667 0.90833333 0.9125 0.91666667 0.92083333 0.925 0.92916667 0.93333333 0.9375 0.94166667 0.94583333 0.95 0.95416667 0.95833333 0.9625 0.96666667 0.97083333 0.975 0.97916667 0.98333333 0.9875 0.99166667 0.99583333 1 1 1 1 1 1
  line L101 (-24.6806, -15.3132) -> (-24.6799, -15.3128)
  arc A50 (-28.5147, -12.1618) -> (-28.1181, -13.0527) centre (0, 0) ccw
  arc A51 (30.9962, -0.4876) -> (30.9962, 0.4876) centre (0, 0) ccw
  spline S47 degree 5 poles (-28.9679, -2.1183) (-28.968, -2.1183) (-28.9682, -2.1183) (-28.9685, -2.1183) (-28.969, -2.1184) (-28.9698, -2.1184) (-28.9706, -2.1185) (-28.9716, -2.1186) (-28.9727, -2.1187) (-28.9739, -2.1188) (-28.9752, -2.1189) (-28.9766, -2.1191) (-28.9781, -2.1192) (-28.9798, -2.1194) (-28.9815, -2.1196) (-28.9833, -2.1198) (-28.9852, -2.12) (-28.9873, -2.1202) (-28.9894, -2.1204) (-28.9916, -2.1207) (-28.9939, -2.121) (-28.9963, -2.1212) (-28.9989, -2.1215) (-29.0015, -2.1219) (-29.0041, -2.1222) (-29.0069, -2.1225) (-29.0098, -2.1229) (-29.0128, -2.1233) (-29.0158, -2.1237) (-29.0189, -2.1241) (-29.0222, -2.1245) (-29.0255, -2.125) (-29.0289, -2.1254) (-29.0323, -2.1259) (-29.0359, -2.1264) (-29.0395, -2.127) (-29.0432, -2.1275) (-29.047, -2.1281) (-29.0509, -2.1286) (-29.0549, -2.1292) (-29.0589, -2.1299) (-29.063, -2.1305) (-29.0672, -2.1312) (-29.0714, -2.1318) (-29.0758, -2.1325) (-29.0802, -2.1332) (-29.0847, -2.134) (-29.0892, -2.1347) (-29.0938, -2.1355) (-29.0985, -2.1363) (-29.1033, -2.1371) (-29.1081, -2.138) (-29.1131, -2.1388) (-29.118, -2.1397) (-29.1231, -2.1406) (-29.1282, -2.1415) (-29.1334, -2.1424) (-29.1386, -2.1434) (-29.1439, -2.1444) (-29.1493, -2.1454) (-29.1547, -2.1464) (-29.1602, -2.1475) (-29.1658, -2.1485) (-29.1714, -2.1496) (-29.1771, -2.1507) (-29.1829, -2.1519) (-29.1887, -2.153) (-29.1946, -2.1542) (-29.2005, -2.1554) (-29.2065, -2.1567) (-29.2126, -2.1579) (-29.2187, -2.1592) (-29.2249, -2.1605) (-29.2311, -2.1618) (-29.2374, -2.1631) (-29.2438, -2.1645) (-29.2502, -2.1659) (-29.2567, -2.1673) (-29.2632, -2.1687) (-29.2698, -2.1702) (-29.2764, -2.1716) (-29.2831, -2.1731) (-29.2899, -2.1747) (-29.2967, -2.1762) (-29.3035, -2.1778) (-29.3104, -2.1794) (-29.3174, -2.181) (-29.3244, -2.1827) (-29.3314, -2.1843) (-29.3386, -2.186) (-29.3457, -2.1877) (-29.3529, -2.1895) (-29.3602, -2.1912) (-29.3675, -2.193) (-29.3749, -2.1948) (-29.3823, -2.1967) (-29.3898, -2.1985) (-29.3973, -2.2004) (-29.4049, -2.2023) (-29.4125, -2.2043) (-29.4202, -2.2062) (-29.4279, -2.2082) (-29.4356, -2.2102) (-29.4434, -2.2123) (-29.4513, -2.2143) (-29.4592, -2.2164) (-29.4671, -2.2185) (-29.4751, -2.2207) (-29.4832, -2.2228) (-29.4912, -2.225) (-29.4994, -2.2272) (-29.5075, -2.2295) (-29.5158, -2.2317) (-29.524, -2.234) (-29.5323, -2.2363) (-29.5407, -2.2387) (-29.5491, -2.241) (-29.5575, -2.2434) (-29.566, -2.2458) (-29.5745, -2.2483) (-29.583, -2.2508) (-29.5917, -2.2533) (-29.6003, -2.2558) (-29.609, -2.2583) (-29.6177, -2.2609) (-29.6265, -2.2635) (-29.6353, -2.2661) (-29.6441, -2.2688) (-29.653, -2.2714) (-29.6619, -2.2741) (-29.6709, -2.2769) (-29.6799, -2.2796) (-29.689, -2.2824) (-29.6981, -2.2852) (-29.7072, -2.288) (-29.7163, -2.2909) (-29.7255, -2.2938) (-29.7348, -2.2967) (-29.7441, -2.2996) (-29.7534, -2.3026) (-29.7627, -2.3056) (-29.7721, -2.3086) (-29.7815, -2.3117) (-29.791, -2.3147) (-29.8005, -2.3178) (-29.81, -2.321) (-29.8196, -2.3241) (-29.8292, -2.3273) (-29.8388, -2.3305) (-29.8485, -2.3337) (-29.8582, -2.337) (-29.868, -2.3403) (-29.8777, -2.3436) (-29.8875, -2.3469) (-29.8974, -2.3503) (-29.9073, -2.3537) (-29.9172, -2.3571) (-29.9271, -2.3606) (-29.9371, -2.364) (-29.9471, -2.3675) (-29.9572, -2.3711) (-29.9673, -2.3746) (-29.9774, -2.3782) (-29.9875, -2.3818) (-29.9977, -2.3855) (-30.0079, -2.3891) (-30.0182, -2.3928) (-30.0284, -2.3965) (-30.0388, -2.4003) (-30.0491, -2.4041) (-30.0595, -2.4079) (-30.0699, -2.4117) (-30.0803, -2.4156) (-30.0907, -2.4194) (-30.1012, -2.4234) (-30.1118, -2.4273) (-30.1223, -2.4313) (-30.1329, -2.4353) (-30.1435, -2.4393) (-30.1541, -2.4433) (-30.1648, -2.4474) (-30.1755, -2.4515) (-30.1862, -2.4557) (-30.197, -2.4598) (-30.2078, -2.464) (-30.2186, -2.4682) (-30.2294, -2.4725) (-30.2403, -2.4767) (-30.2512, -2.481) (-30.2621, -2.4854) (-30.2731, -2.4897) (-30.2841, -2.4941) (-30.2951, -2.4985) (-30.3061, -2.503) (-30.3172, -2.5074) (-30.3283, -2.5119) (-30.3394, -2.5165) (-30.3506, -2.521) (-30.3617, -2.5256) (-30.3729, -2.5302) (-30.3841, -2.5348) (-30.3954, -2.5395) (-30.4067, -2.5442) (-30.418, -2.5489) (-30.4293, -2.5537) (-30.4407, -2.5584) (-30.452, -2.5632) (-30.4634, -2.5681) (-30.4749, -2.5729) (-30.4863, -2.5778) (-30.4978, -2.5827) (-30.5093, -2.5877) (-30.5208, -2.5927) (-30.5324, -2.5977) (-30.5439, -2.6027) (-30.5555, -2.6077) (-30.5672, -2.6128) (-30.5788, -2.6179) (-30.5905, -2.6231) (-30.6022, -2.6283) (-30.6139, -2.6335) (-30.6256, -2.6387) (-30.6374, -2.6439) (-30.6492, -2.6492) (-30.661, -2.6545) (-30.6728, -2.6599) (-30.6847, -2.6653) (-30.6966, -2.6707) (-30.7085, -2.6761) (-30.7204, -2.6815) (-30.7323, -2.687) (-30.7443, -2.6925) (-30.7563, -2.6981) (-30.7683, -2.7036) (-30.7803, -2.7092) (-30.7924, -2.7149) (-30.8044, -2.7205) (-30.8165, -2.7262) (-30.8287, -2.7319) (-30.8408, -2.7376) (-30.853, -2.7434) (-30.8627, -2.748) (-30.87, -2.7515) (-30.8749, -2.7539) (-30.8773, -2.755) knots 0 0 0 0 0 0 0.00416667 0.00833333 0.0125 0.01666667 0.02083333 0.025 0.02916667 0.03333333 0.0375 0.04166667 0.04583333 0.05 0.05416667 0.05833333 0.0625 0.06666667 0.07083333 0.075 0.07916667 0.08333333 0.0875 0.09166667 0.09583333 0.1 0.10416667 0.10833333 0.1125 0.11666667 0.12083333 0.125 0.12916667 0.13333333 0.1375 0.14166667 0.14583333 0.15 0.15416667 0.15833333 0.1625 0.16666667 0.17083333 0.175 0.17916667 0.18333333 0.1875 0.19166667 0.19583333 0.2 0.20416667 0.20833333 0.2125 0.21666667 0.22083333 0.225 0.22916667 0.23333333 0.2375 0.24166667 0.24583333 0.25 0.25416667 0.25833333 0.2625 0.26666667 0.27083333 0.275 0.27916667 0.28333333 0.2875 0.29166667 0.29583333 0.3 0.30416667 0.30833333 0.3125 0.31666667 0.32083333 0.325 0.32916667 0.33333333 0.3375 0.34166667 0.34583333 0.35 0.35416667 0.35833333 0.3625 0.36666667 0.37083333 0.375 0.37916667 0.38333333 0.3875 0.39166667 0.39583333 0.4 0.40416667 0.40833333 0.4125 0.41666667 0.42083333 0.425 0.42916667 0.43333333 0.4375 0.44166667 0.44583333 0.45 0.45416667 0.45833333 0.4625 0.46666667 0.47083333 0.475 0.47916667 0.48333333 0.4875 0.49166667 0.49583333 0.5 0.50416667 0.50833333 0.5125 0.51666667 0.52083333 0.525 0.52916667 0.53333333 0.5375 0.54166667 0.54583333 0.55 0.55416667 0.55833333 0.5625 0.56666667 0.57083333 0.575 0.57916667 0.58333333 0.5875 0.59166667 0.59583333 0.6 0.60416667 0.60833333 0.6125 0.61666667 0.62083333 0.625 0.62916667 0.63333333 0.6375 0.64166667 0.64583333 0.65 0.65416667 0.65833333 0.6625 0.66666667 0.67083333 0.675 0.67916667 0.68333333 0.6875 0.69166667 0.69583333 0.7 0.70416667 0.70833333 0.7125 0.71666667 0.72083333 0.725 0.72916667 0.73333333 0.7375 0.74166667 0.74583333 0.75 0.75416667 0.75833333 0.7625 0.76666667 0.77083333 0.775 0.77916667 0.78333333 0.7875 0.79166667 0.79583333 0.8 0.80416667 0.80833333 0.8125 0.81666667 0.82083333 0.825 0.82916667 0.83333333 0.8375 0.84166667 0.84583333 0.85 0.85416667 0.85833333 0.8625 0.86666667 0.87083333 0.875 0.87916667 0.88333333 0.8875 0.89166667 0.89583333 0.9 0.90416667 0.90833333 0.9125 0.91666667 0.92083333 0.925 0.92916667 0.93333333 0.9375 0.94166667 0.94583333 0.95 0.95416667 0.95833333 0.9625 0.96666667 0.97083333 0.975 0.97916667 0.98333333 0.9875 0.99166667 0.99583333 1 1 1 1 1 1
  arc A52 (29.3284, -10.0421) -> (29.6298, -9.1146) centre (0, 0) ccw